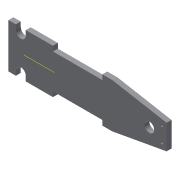
# Autodesk Inventor part: pcb
Saved by Autodesk Inventor 2022 (Build 260148000, 148)
## iProperties
Shininess: 64.0
Length Units: 11269
Angle Units: 11279
Time Units: 11290
Mass Units: 11283
Length Display Precision: 3
Angle Display Precision: 2
Created: 2002-02-13
Part Number: pcb
Document SubType Name: Modeling
Designer: Administrator
Density: 1 g/cm^3
Material: Generic
Appearance: Default
Density: 0.0
Volumn: 0.0
Area: 0.0
PropertySet Name: Model Information
Control State: 0
Master: False
Checked Out: False
Author: Administrator
Autodesk Inventor part; units mm, degrees
ref_plane "YZ Plane" through (0, 0, 0) normal (1, 0, 0) x (0, 1, 0)
ref_plane "XZ Plane" through (0, 0, 0) normal (0, 1, 0) x (-1, 0, 0)
ref_plane "XY Plane" through (0, 0, 0) normal (0, 0, 1) x (1, 0, 0)
sketch "Sketch1" plane through (0, 0, 0) normal (0, 0, 1) x (1, 0, 0)
  line L0 (8.2169, 9.2649) -> (8.2169, -5.0211)
  line L1 (8.2169, -5.0211) -> (41.5544, -5.0211)
  line L2 (41.5544, -5.0211) -> (59.0169, -1.8469)
  line L3 (59.0169, -1.8469) -> (59.0169, 6.0906)
  line L4 (59.0169, 6.0906) -> (41.5544, 9.2649)
  line L5 (41.5544, 9.2649) -> (8.2169, 9.2649)
  line L6 (59.0169, 2.1219) -> (8.2169, 2.1219) construction
  line L7 (3.1369, 0) -> (74.2569, 0) projected
  line L8 (0, 13.5507) -> (0, -6.4497) projected
  dimension "d1" = 33.3375
  dimension "d2" = 50.8
  dimension "d3" = 7.9375
  dimension "d92" = 7.143
  dimension "d93" = 2.1218
  dimension "d94" = 8.2169
  constraints: 14 end point, 2 equal length, 2 midpoint, 2 parallel, 1 horizontal, 1 perpendicular, 1 vertical
  measures "d1" distance of L4.end L0.start
  measures "d2" horizontal distance of L3.end L0.start
  measures "d3" distance of L2.end L3.end
  measures "d92" distance between parallel lines of L5 L6
  measures "d93" distance between parallel lines of L7 L6
  measures "d94" distance between parallel lines of L8 L0
extrude "Extrusion1" add sketch "Sketch1" along normal blind 1.5875
sketch "Sketch12" plane through (0, 0, 1.5875) normal (0, 0, 1) x (1, 0, 0)
  line L0 (8.2169, 9.2649) -> (41.5544, 9.2649) projected
  line L1 (8.2169, -5.0211) -> (8.2169, 9.2649) projected
  line L2 (22.5044, 9.2649) -> (38.3794, 9.2649)
  line L3 (38.3794, 9.2649) -> (38.3794, 7.6774)
  line L4 (38.3794, 7.6774) -> (22.5044, 7.6774)
  line L5 (22.5044, 7.6774) -> (22.5044, 9.2649)
  dimension "d63" = 15.875
  dimension "d64" = 1.5875
  dimension "d65" = 14.2875
  constraints: 8 end point, 2 parallel, 1 collinear, 1 horizontal, 1 perpendicular
  measures "d63" distance of L2.start L2.end
  measures "d64" distance of L4.end L2.start
  measures "d65" distance between parallel lines of L5 L1
extrude "Extrusion12" cut sketch "Sketch12" against normal through all
sketch "Sketch13" plane through (0, 0, 1.5875) normal (0, 0, 1) x (1, 0, 0)
  line L0 (8.2169, 9.2649) -> (22.5044, 9.2649) projected
  line L1 (38.3794, 7.6774) -> (22.5044, 7.6774) projected
  line L2 (10.5981, 9.2649) -> (10.5981, 7.6774)
  arc A0 (10.5981, 7.6774) -> (13.7731, 7.6774) centre (12.1856, 7.6774) ccw
  line L3 (13.7731, 7.6774) -> (13.7731, 9.2649)
  line L4 (22.5044, 7.6774) -> (22.5044, 9.2649) projected
  line L5 (8.2169, -5.0211) -> (8.2169, 9.2649) projected
  line L6 (41.5544, -5.0211) -> (8.2169, -5.0211) projected
  line L7 (59.0169, -1.8469) -> (41.5544, -5.0211) projected
  line L8 (59.0169, 6.0906) -> (59.0169, -1.8469) projected
  line L9 (41.5544, 9.2649) -> (59.0169, 6.0906) projected
  line L10 (38.3794, 9.2649) -> (41.5544, 9.2649) projected
  line L11 (38.3794, 9.2649) -> (38.3794, 7.6774) projected
  dimension "d68" = 1.5875
  dimension "d69" = 1.5875
  dimension "d70" = 3.9688
  constraints: 4 end point, 2 perpendicular, 2 point on circle, 2 point on line, 2 tangent, 1 centre point
  measures "d68" radius of A0
  measures "d69" vertical distance of L0.start A0.centre
  measures "d70" horizontal distance of L0.start A0.centre
extrude "Extrusion13" cut sketch "Sketch13" against normal blind 25.4 contours L0 L3 A0 L2
ref_plane "Work Plane5" through (22.5044, 2.1211, 1.5875) normal (0, 1, 0) x (1, 0, 0)
mirror "Mirror2" about plane through (22.5044, 2.1211, 1.5875) normal (0, 1, 0) of "Extrusion12", "Extrusion13"
sketch "Sketch14" plane through (0, 0, 1.5875) normal (0, 0, 1) x (1, 0, 0)
  line L0 (3.1369, 2.1211) -> (74.2569, 2.1211) projected
  line L1 (13.7731, 9.2649) -> (22.5044, 9.2649) projected
  line L2 (8.2169, -5.0211) -> (8.2169, 9.2649) projected
  point P0 (53.4606, 2.1219)
  dimension "d95" = 45.2437
  dimension "d96" = 7.143
  measures "d95" distance from line of L2 point (53.461, 2.122)
  measures "d96" distance from line of L1 point (53.461, 2.122)
hole "Hole1" at (53.4606, 2.1219, 1.5875) direction (0, 0, -1) diameter 3.175 end through all
sketch "Sketch15" plane through (0, 0, 1.5875) normal (0, 0, 1) x (1, 0, 0)
  line L0 (10.5981, -5.0211) -> (10.5981, -3.4351) projected
  line L1 (59.0169, 6.0906) -> (57.4294, 4.5031)
  line L2 (57.4294, 4.5031) -> (57.4294, -0.2594)
  line L3 (57.4294, -0.2594) -> (59.0169, -1.8469)
  dimension "d82" = 4.7625
  dimension "d84" = 1.5875
  constraints: 6 end point, 1 parallel, 1 perpendicular
  measures "d82" distance of L1.end L2.end
  measures "d84" horizontal distance of L2.end L3.end
hole "Hole2" at (57.4294, 4.5031, 1.5875) at (57.4294, -0.2594, 1.5875) direction (0, 0, -1) diameter 0.762 end through all
equation "\"d96\" = d92"
body "Solid1"
